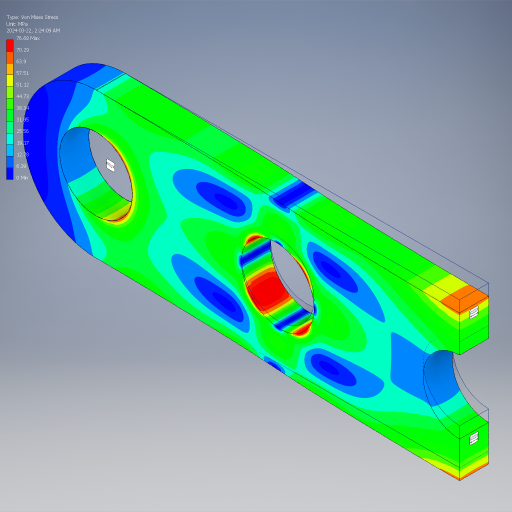
# Autodesk Inventor part: CE-10.2.1.2
Saved by Autodesk Inventor 2024 (Build 280153000, 153)
## iProperties
Created: 2024-03-22
Part Number: CE-10.2.1.2
Material: Aluminum 6061
Document SubType Name: Modeling
Designer: Alex
Density: 2.7 g/cm^3
Appearance: Aluminum - Flat
Author: Alex
Autodesk Inventor part; units mm, degrees
ref_plane "YZ Plane" through (0, 0, 0) normal (1, 0, 0) x (0, 1, 0)
ref_plane "XZ Plane" through (0, 0, 0) normal (0, 1, 0) x (-1, 0, 0)
ref_plane "XY Plane" through (0, 0, 0) normal (0, 0, 1) x (1, 0, 0)
sketch "Sketch1" plane through (0, 0, 0) normal (0, 0, 1) x (1, 0, 0)
  line L0 (-250, 0) -> (0, 0) construction
  line L1 (-250, -50) -> (0, -50)
  line L2 (0, 50) -> (-250, 50)
  arc A0 (-250, 50) -> (-250, -50) centre (-250, 0) ccw
  line L3 (0, 50) -> (0, -50)
  circle A1 centre (-250, 0) radius 25
  circle A2 centre (-125, 0) radius 25
  circle A3 centre (0, 0) radius 25
  point P0 (-125, 0)
  point P1 (0, -25)
  point P2 (0, 25)
  dimension "d2" = 250
  dimension "d3" = 50
  dimension "d4" = 50
  dimension "d6" = 125
  dimension "d7" = 125
  constraints: 10 end point, 4 centre point, 4 midpoint, 2 coincident, 2 equal radius, 2 point on circle, 2 tangent, 1 horizontal, 1 parallel, 1 point on line, 1 vertical
  measures "d2" distance of L2.start L2.end
  measures "d3" radius of A0
  measures "d4" diameter of A1
  measures "d6" distance of A2.centre L0.start
  measures "d7" distance of point (0, 0) point (-125, 0)
extrude "Extrusion1" add sketch "Sketch1" along normal mid plane 20 contours A0 L2 L3 A3 L1
body "Solid1"
